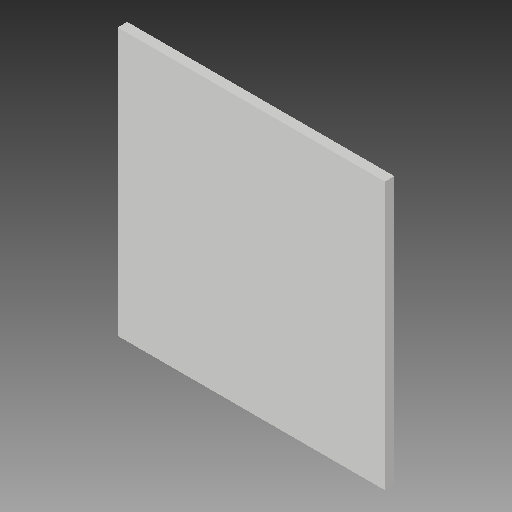
# Autodesk Inventor part: Sciana_168x168
Saved by Autodesk Inventor 2018 (Build 220112000, 112)
## iProperties
Created: 2018-10-19
Part Number: Sciana_168x168
Material: Ogólny
Document SubType Name: Modeling
Designer: EWA
Density: 1 g/cm^3
Appearance: Domyślna
Author: EWA
Autodesk Inventor part; units mm, degrees
ref_plane "YZ Plane" through (0, 0, 0) normal (1, 0, 0) x (0, 1, 0)
ref_plane "XZ Plane" through (0, 0, 0) normal (0, 1, 0) x (-1, 0, 0)
ref_plane "XY Plane" through (0, 0, 0) normal (0, 0, 1) x (1, 0, 0)
sketch "Szkic1" plane through (0, 0, 0) normal (0, 0, 1) x (1, 0, 0)
  line L0 (0, 0) -> (168, 0)
  line L1 (168, 0) -> (168, 168)
  line L2 (168, 168) -> (0, 168)
  line L3 (0, 168) -> (0, 0)
  dimension "d0" = 168
  dimension "d1" = 168
  constraints: 8 end point, 2 parallel, 1 horizontal, 1 perpendicular
  measures "d0" distance of L2.end L1.end
  measures "d1" distance of L1.end L0.end
extrude "Wyciągnięcie proste1" add sketch "Szkic1" along normal blind 6
